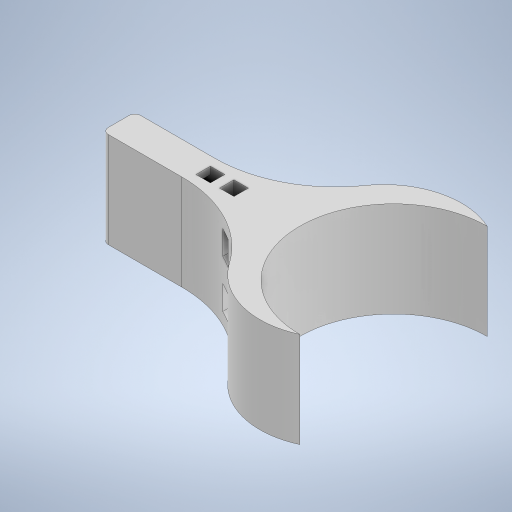
# Autodesk Inventor part: ReedHolder
Saved by Autodesk Inventor 2023 (Build 270158000, 158)
## iProperties
Created: 2023-06-06
Part Number: ReedHolder
Material: Generic
Document SubType Name: Modeling
Designer: Joshua
Density: 1 g/cm^3
Appearance: Default
Author: Joshua
Autodesk Inventor part; units mm, degrees
ref_plane "YZ Plane" through (0, 0, 0) normal (1, 0, 0) x (0, 1, 0)
ref_plane "XZ Plane" through (0, 0, 0) normal (0, 1, 0) x (-1, 0, 0)
ref_plane "XY Plane" through (0, 0, 0) normal (0, 0, 1) x (1, 0, 0)
sketch "Sketch1" plane through (0, 0, 0) normal (0, 1, 0) x (-1, 0, 0)
  line L0 (0, 0) -> (29.21, 0)
  line L1 (29.21, 0) -> (29.21, -6.858)
  line L2 (29.21, -6.858) -> (0, -6.858)
  line L3 (0, -6.858) -> (0, 0)
  line L4 (0, 0) -> (-3.81, 0)
  line L5 (-3.81, 0) -> (-3.81, -6.858)
  line L6 (-3.81, -6.858) -> (0, -6.858)
  line L7 (0, -6.858) -> (0, 0)
  circle A0 centre (-28.575, -3.429) radius 19.685
  circle A1 centre (-28.575, -3.429) radius 24.765
  arc A2 (-8.3079, 10.803) -> (12.4788, 0) centre (12.4788, 25.4) ccw
  arc A3 (12.4788, -6.858) -> (-8.3079, -17.661) centre (12.4788, -32.258) ccw
  line L8 (-28.575, -3.429) -> (-28.575, 21.336)
  line L9 (-28.575, -3.429) -> (-3.81, -3.429) construction
  line L10 (-28.575, -3.429) -> (-28.575, -28.194)
  arc A4 (-8.3079, 10.803) -> (-28.575, 16.256) centre (-21.7065, 1.3942) ccw
  arc A5 (-28.575, -23.114) -> (-8.3079, -17.661) centre (-21.7065, -8.2522) ccw
  point P0 (0, -3.429)
  dimension "d0" = 29.21
  dimension "d1" = 6.858
  dimension "d4" = 3.81
  dimension "d5" = 39.37
  dimension "d6" = 6.858
  dimension "d7" = 5.08
  dimension "d8" = 25.4
  dimension "d9" = 25.4
  dimension "d10" = 180
  dimension "d11" = 90
  dimension "d12" = 90
  constraints: 22 end point, 15 point on circle, 6 centre point, 6 tangent, 4 parallel, 4 point on line, 2 horizontal, 2 midpoint, 2 perpendicular, 1 coincident, 1 horizontal alignment
  measures "d0" distance of L1.end L2.end
  measures "d1" distance of L0.end L1.end
  measures "d4" distance of L6.end L5.end
  measures "d5" diameter of A0
  measures "d6" distance of L4.end L5.end
  measures "d7" radial gap between concentric circles of A1 A0
  measures "d8" radius of A2
  measures "d9" radius of A3
  measures "d10" angle of L8 L10
  measures "d11" angle of L9 L10
  measures "d12" angle of L9 L8
extrude "Extrusion1" add sketch "Sketch1" along normal blind 20.066 contours L4 L5 A1 A2 L0 | L0 L1 L2 L3 | L3 L6 L5 L4 | L2 A3 A1 L5 L6 | A1 A5 A0 A4
sketch "Sketch3" plane through (-29.21, 0, 0) normal (0, 0, 1) x (1, 0, 0)
  line L0 (0, 0) -> (16.7312, 0) projected
  line L1 (16.7312, 0) -> (16.7312, 20.066) projected
  line L2 (0, 20.066) -> (16.7312, 20.066) projected
  line L3 (0, 0) -> (0, 20.066) projected
  line L4 (16.7312, 0) -> (37.5179, 0) projected
  line L5 (37.5179, 0) -> (37.5179, 20.066) projected
  line L6 (16.7312, 20.066) -> (37.5179, 20.066) projected
  line L7 (16.7312, 0) -> (16.7312, 20.066) projected
  line L8 (37.5179, 0) -> (57.785, 0) projected
  line L9 (57.785, 0) -> (57.785, 20.066) projected
  line L10 (37.5179, 20.066) -> (57.785, 20.066) projected
  line L11 (37.5179, 0) -> (37.5179, 20.066) projected
  line L12 (0, 0) -> (0, 20.066) projected
  line L13 (0, 10.033) -> (29.21, 10.033) construction
  line L14 (16.7312, 20.066) -> (37.5179, 20.066) projected
  line L15 (29.21, 20.066) -> (29.21, 0) construction
  line L16 (16.7312, 0) -> (37.5179, 0) projected
  line L17 (27.94, 12.5095) -> (30.48, 12.5095)
  line L18 (30.48, 12.5095) -> (30.48, 17.5895)
  line L19 (30.48, 17.5895) -> (27.94, 17.5895)
  line L20 (27.94, 17.5895) -> (27.94, 12.5095)
  line L21 (27.94, 7.5565) -> (30.48, 7.5565)
  line L22 (30.48, 7.5565) -> (30.48, 2.4765)
  line L23 (30.48, 2.4765) -> (27.94, 2.4765)
  line L24 (27.94, 2.4765) -> (27.94, 7.5565)
  point P0 (29.21, 0)
  point P1 (29.21, 12.5095)
  dimension "d13" = 29.21
  dimension "d14" = 2.54
  dimension "d15" = 5.08
  dimension "d16" = 2.4765
  dimension "d17" = 2.4765
  constraints: 20 end point, 4 midpoint, 4 point on line, 4 symmetric about line, 3 perpendicular, 2 parallel, 1 horizontal
  measures "d13" distance of L13.start L13.end
  measures "d14" distance of L19.end L18.end
  measures "d15" distance of L18.end L17.end
  measures "d16" distance between parallel lines of L13 L17
  measures "d17" distance between parallel lines of L6 L19
extrude "Extrusion2" cut sketch "Sketch3" along normal through all both and the other way through all contours L20 L19 L18 L17 | L21 L22 L23 L24
sketch "Sketch4" plane through (-29.21, 0, 0) normal (0, 0, 1) x (1, 0, 0)
  line L0 (0, 20.066) -> (16.7312, 20.066) projected
  line L1 (0, 0) -> (16.7312, 0) projected
  line L2 (0, 0) -> (0, 20.066) projected
  line L3 (0, 18.542) -> (2.794, 18.542)
  line L4 (2.794, 18.542) -> (2.794, 1.524)
  line L5 (2.794, 1.524) -> (0, 1.524)
  line L6 (0, 1.524) -> (0, 18.542)
  line L7 (0, 10.033) -> (17.78, 10.033) construction
  line L8 (2.794, 18.542) -> (17.78, 18.542)
  line L9 (17.78, 18.542) -> (17.78, 15.494)
  line L10 (17.78, 15.494) -> (2.794, 15.494)
  line L11 (2.794, 15.494) -> (2.794, 18.542)
  line L12 (16.7312, 20.066) -> (37.5179, 20.066) projected
  line L13 (17.78, 15.494) -> (20.828, 15.494)
  line L14 (20.828, 15.494) -> (20.828, 20.066)
  line L15 (20.828, 20.066) -> (17.78, 20.066)
  line L16 (17.78, 20.066) -> (17.78, 15.494)
  line L17 (2.794, 1.524) -> (22.733, 1.524)
  line L18 (22.733, 1.524) -> (22.733, 4.572)
  line L19 (22.733, 4.572) -> (2.794, 4.572)
  line L20 (2.794, 4.572) -> (2.794, 1.524)
  line L21 (22.733, 1.524) -> (25.781, 1.524)
  line L22 (25.781, 1.524) -> (25.781, 20.066)
  line L23 (25.781, 20.066) -> (22.733, 20.066)
  line L24 (22.733, 20.066) -> (22.733, 1.524)
  point P0 (29.21, 0)
  point P1 (17.78, 17.018)
  point P2 (2.794, 4.572)
  point P3 (2.794, 15.494)
  point P4 (17.78, 18.542)
  dimension "d25" = 2.794
  dimension "d26" = 17.018
  dimension "d27" = 1.524
  dimension "d28" = 1.524
  dimension "d29" = 17.78
  dimension "d30" = 3.048
  dimension "d31" = 3.048
  dimension "d32" = 1.905
  dimension "d33" = 3.048
  dimension "d34" = 3.048
  constraints: 42 end point, 10 parallel, 6 horizontal, 5 perpendicular, 3 midpoint, 2 point on line, 1 vertical alignment
  measures "d25" distance of L4.end L5.end
  measures "d26" distance of L3.end L4.end
  measures "d27" distance between parallel lines of L1 L5
  measures "d28" distance between parallel lines of L0 L3
  measures "d29" distance of L7.start L7.end
  measures "d30" distance between parallel lines of L8 L10
  measures "d31" distance of L15.end L14.end
  measures "d32" distance between parallel lines of L14 L18
  measures "d33" distance of L23.end L22.end
  measures "d34" distance between parallel lines of L17 L19
extrude "Extrusion3" cut sketch "Sketch4" against normal blind 4.953 contours L3 L4 L5 L2 | L12 L14 L13 L9 L16 | L8 L9 L10 L4 | L4 L19 L18 L17 | L12 L22 L21 L18 L24
sketch "Sketch5" plane through (-26.416, 4.572, 0) normal (0, 0, 1) x (1, 0, 0)
  line L0 (-2.794, 13.97) -> (13.9372, 13.97) projected
  line L1 (13.9372, 10.922) -> (0, 10.922) projected
  line L2 (13.9372, 10.922) -> (13.9372, 13.97) projected
  line L3 (-2.794, -3.048) -> (-2.794, 13.97) projected
  line L4 (0, 10.922) -> (0, 0) projected
  line L5 (13.9372, -3.048) -> (-2.794, -3.048) projected
  line L6 (0, 0) -> (13.9372, 0) projected
  line L7 (13.9372, -3.048) -> (13.9372, 0) projected
  line L8 (13.9372, 10.922) -> (13.9372, 13.97) projected
  line L9 (14.986, 13.97) -> (13.9372, 13.97) projected
  line L10 (14.986, 15.494) -> (14.986, 13.97) projected
  line L11 (18.034, 15.494) -> (14.986, 15.494) projected
  line L12 (18.034, 10.922) -> (18.034, 15.494) projected
  line L13 (13.9372, 10.922) -> (18.034, 10.922) projected
  line L14 (13.9372, -3.048) -> (13.9372, 0) projected
  line L15 (19.939, 0) -> (13.9372, 0) projected
  line L16 (19.939, 15.494) -> (19.939, 0) projected
  line L17 (22.987, 15.494) -> (19.939, 15.494) projected
  line L18 (22.987, -3.048) -> (22.987, 15.494) projected
  line L19 (13.9372, -3.048) -> (22.987, -3.048) projected
  point P0 (26.416, -4.572)
extrude "Extrusion4" add sketch "Sketch5" against normal blind 1.905
fillet "Fillet1" radius 1.27 2 edges at (-29.21, 10.033, 0) (-29.21, 10.033, -6.858)
equation "\"d6\" = d1"
equation "\"d9\" = d8"
equation "\"d11\" = d12"
equation "\"d16\" = d17"
equation "\"d27\" = d28"
body "Solid1"
